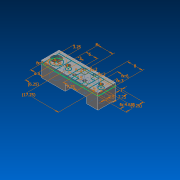
# Autodesk Inventor part: tac switch body
Saved by Autodesk Inventor 2015 (Build 190159000, 159)
## iProperties
Created: 2017-03-16
Part Number: tac switch body
Material: Generic
Document SubType Name: Modeling
Designer: ZigZagJoe
Density: 1 g/cm^3
Appearance: Default
Author: ZigZagJoe
Autodesk Inventor part; units mm, degrees
ref_plane "YZ Plane" through (0, 0, 0) normal (1, 0, 0) x (0, 1, 0)
ref_plane "XZ Plane" through (0, 0, 0) normal (0, 1, 0) x (-1, 0, 0)
ref_plane "XY Plane" through (0, 0, 0) normal (0, 0, 1) x (1, 0, 0)
sketch "Sketch1" plane through (0, 0, 0) normal (0, 0, 1) x (1, 0, 0)
  line L0 (-7.1784, -0.1841) -> (0.0716, -0.1841)
  line L1 (0.0716, -0.1841) -> (0.0716, -7.4341)
  line L2 (0.0716, -7.4341) -> (-7.1784, -7.4341)
  line L3 (-7.1784, -7.4341) -> (-7.1784, -0.1841)
  line L4 (-7.1784, -2.1841) -> (-5.1784, -2.1841)
  line L5 (-5.1784, -2.1841) -> (-5.1784, -0.1841)
  line L6 (-1.9284, -0.1841) -> (-1.9284, -2.1841)
  line L7 (-1.9284, -2.1841) -> (0.0716, -2.1841)
  line L8 (-7.1784, -5.4341) -> (-5.1784, -5.4341)
  line L9 (-5.1784, -5.4341) -> (-5.1784, -7.4341)
  line L10 (-1.9284, -5.4341) -> (0.0716, -5.4341)
  line L11 (-1.9284, -5.4341) -> (-1.9284, -7.4341)
  line L12 (8.0716, 0.8159) -> (8.0716, -8.4341)
  line L13 (-15.1784, -8.4341) -> (-15.1784, 0.8159)
  circle A0 centre (-12.1784, -3.8091) radius 1.25
  circle A1 centre (5.0716, -3.8091) radius 1.25
  line L14 (-15.1784, 0.8159) -> (-9.1784, 0.8159)
  line L15 (-9.1784, 0.8159) -> (-9.1784, -8.4341)
  line L16 (-9.1784, -8.4341) -> (-15.1784, -8.4341)
  line L17 (-15.1784, -8.4341) -> (-15.1784, 0.8159)
  line L18 (8.0716, 0.8159) -> (2.0716, 0.8159)
  line L19 (2.0716, 0.8159) -> (2.0716, -8.4341)
  line L20 (2.0716, -8.4341) -> (8.0716, -8.4341)
  line L21 (8.0716, -8.4341) -> (8.0716, 0.8159)
  line L22 (-9.1784, 0.8159) -> (2.0716, 0.8159)
  line L23 (-9.1784, -8.4341) -> (2.0716, -8.4341)
  line L24 (-15.1784, 0.8159) -> (-21.6784, 0.8159)
  line L25 (-21.6784, 0.8159) -> (-21.6784, -8.4341)
  line L26 (-21.6784, -8.4341) -> (-15.1784, -8.4341)
  line L27 (-15.1784, -8.4341) -> (-15.1784, 0.8159)
  circle A2 centre (-18.4284, -3.8091) radius 2.625
  point P0 (0, 0)
  dimension "d0" = 7.25
  dimension "d1" = 7.25
  dimension "d2" = 2
  dimension "d3" = 2
  dimension "d4" = 2
  dimension "d5" = 2
  dimension "d6" = 8
  dimension "d7" = 8
  dimension "d10" = 2.5
  dimension "d11" = 2.5
  dimension "d12" = 6
  dimension "d13" = 6
  dimension "d14" = 3
  dimension "d15" = 3
  dimension "d23" = 1
  dimension "d24" = 1
  dimension "d25" = 9.25
  dimension "d26" = 4.625
  dimension "d27" = 4.625
  dimension "d28" = 17.25
  dimension "d29" = 5.25
  dimension "d30" = 3.25
  dimension "d31" = 6.5
  dimension "d33" = 6.25
  constraints: 56 end point, 15 point on line, 12 parallel, 6 horizontal, 6 perpendicular, 3 centre point
  measures "d0" distance of L1.end L2.end
  measures "d1" distance of L0.end L1.end
  measures "d2" distance of L4.start L4.end
  measures "d3" distance of L4.end L5.end
  measures "d4" distance of L6.end L7.end
  measures "d5" distance of L10.start L11.end
  measures "d6" distance between parallel lines of L13 L3
  measures "d7" distance between parallel lines of L12 L1
  measures "d10" diameter of A0
  measures "d11" diameter of A1
  measures "d12" distance between parallel lines of L13 L15
  measures "d13" distance between parallel lines of L12 L19
  measures "d14" distance from line of L13 A0.centre
  measures "d15" distance from line of L12 A1.centre
  measures "d23" distance between parallel lines of L22 L0
  measures "d24" distance between parallel lines of L23 L2
  measures "d25" distance between parallel lines of L18 L20
  measures "d26" distance from line of L20 A1.centre
  measures "d27" distance from line of L16 A0.centre
  measures "d28" distance of A0.centre A1.centre
  measures "d29" diameter of A2
  measures "d30" distance from line of L25 A2.centre
  measures "d31" distance of L25.end L26.end
  measures "d33" distance of A0.centre A2.centre
extrude "Extrusion1" add sketch "Sketch1" along normal blind 1.5 contours L0 L6 L7 L1 L10 L11 L2 L9 L8 L3 L4 L5 | L12 L20 L19 L18 | L19 L23 L15 L22 | L15 L16 L13 L14 | L13 L26 L25 L24
extrude "Extrusion2" add sketch "Sketch1" against normal blind 3.5
extrude "Extrusion3" add sketch "Sketch1" against normal blind 6.5 contours L12 L20 L19 L18 | L15 L16 L13 L14 | L13 L26 L25 L24
equation "\"d2\" = d5"
equation "\"d3\" = d5"
equation "\"d4\" = d5"
equation "\"d13\" = d12"
equation "\"d15\" = d14"
equation "\"d26\" = 0.5 * d25"
equation "\"d27\" = d26"
body "Solid1"
